Autodesk Fusion 360 part; units mm, degrees
note: some values were not read from the file. Set by a fixed rule: which sketch regions a step uses.
(part 2 of 2)
  constraint tangent L244 A250
  constraint tangent L243 A251
  constraint tangent L250 A251
  constraint tangent L251 A252
  constraint tangent L243 A252
  constraint tangent L242 A253
  constraint tangent L251 A253
  constraint tangent L242 A254
  constraint tangent L241 A254
  constraint tangent L241 A255
  constraint tangent L240 A255
  constraint tangent L240 A256
  constraint tangent L239 A256
  constraint tangent L239 A257
  constraint tangent L238 A257
  constraint perpendicular L104 L253
  constraint coincident L216 L253.start
  constraint tangent L229 A258
  constraint tangent L106 A259
  constraint tangent L253 A259
  constraint tangent L229 A260
  constraint tangent L106 A260
  constraint tangent L252 A261
  constraint tangent L252 A262
  measures "d1" diameter of A0
  measures "d2" diameter of A1
  measures "d3" diameter of A2
  measures "d4" diameter of A3
  measures "d5" diameter of A4
  measures "d9" diameter of A111
  measures "d12" diameter of A112
extrude "Extrude1" add sketch "mriya-bumper-fdm" along normal blind 10.5 contours L181 L182 L207 A214 L208 A215 L209 A216 L210 A217 L211 A218 L212 A219 L213 A220 L214 A221 L215 A222 L216 L217 A224 L218 A225 L219 A226 L220 A227 L221 A228 L222 A229 L223 A230 L224 A231 L225 A232 L226 A233 L227 A234 L228 A235 L230 L231 L232 L233 L234 L235 L236 L237 L238 L239 L240 L241 L242 L243 L244 L245 L246 L247 L248 L249 L250 L251 A236 A237 A239 A240 A241 A242 A243 A244 A245 A246 A247 A248 A249 A250 A251 A252 A253 A254 A255 A256 A257 makes body 1
extrude "Extrude2" add sketch "mriya-bumper-fdm" along normal blind 17 contours L181 L182 L216 A223 L217 L245 L246 A238 bodies 1
extrude "Extrude3" add sketch "mriya-bumper-fdm" along normal blind 2 from surface at 1.7 contours L106 L207 A214 L208 A215 L209 A216 L210 A217 L211 A218 L212 A219 L213 A220 L214 A221 L215 A222 L216 L217 A224 L218 A225 L219 A226 L220 A227 L221 A228 L222 A229 L223 A230 L224 A231 L225 A232 L226 A233 L227 A234 L228 A235 L229 L252 A258 A259 A260 A261 A262 | L106 L216 A223 L217 L229 A258 A259 A260 | L216 L252 A261 A262 | A114 | A115 | A116 | A117 bodies 1
extrude "Extrude6" add sketch "mriya-bumper-fdm" along normal blind 1 from surface at 14.3 contours L106 L216 A223 L217 L229 A258 A259 A260 bodies 1
extrude "Extrude12" add sketch "mriya-bumper-fdm" along normal blind 1 from surface at 7.7 contours L216 L252 A261 A262 bodies 1
sketch "power-switch" plane through (-4.4, 0, 0) normal (1, 0, 0) x (0, 1, 0)
  line L0 (1.7932, 0) -> (76.6932, 0)
  line L1 (76.6932, 0) -> (76.6932, 17)
  line L2 (76.6932, 17) -> (19.2932, 17)
  line L3 (19.2932, 17) -> (19.2932, 10.5)
  line L4 (19.2932, 10.5) -> (1.7932, 10.5)
  line L5 (1.7932, 10.5) -> (1.7932, 0)
  line L6 (25.6932, 5.4) -> (25.6932, 8.35)
  line L7 (36.0932, 5.4) -> (25.6932, 5.4)
  arc A0 (37.3932, 4.05) -> (37.7932, 4.45) centre (37.3932, 4.45) ccw
  arc A1 (24.3932, 9.7) -> (23.9932, 9.3) centre (24.3932, 9.3) ccw
  line L8 (23.9932, 4.45) -> (23.9932, 9.3)
  line L9 (25.6932, 8.35) -> (36.0932, 8.35)
  arc A2 (23.9932, 4.45) -> (24.3932, 4.05) centre (24.3932, 4.45) ccw
  line L10 (37.7932, 9.3) -> (37.7932, 4.45)
  line L11 (37.3932, 4.05) -> (24.3932, 4.05)
  line L12 (24.3932, 9.7) -> (37.3932, 9.7)
  line L13 (36.0932, 8.35) -> (36.0932, 5.4)
  arc A3 (37.7932, 9.3) -> (37.3932, 9.7) centre (37.3932, 9.3) ccw
  constraint perpendicular L6 L7
  constraint vertical L6
  constraint perpendicular L6 L9
  constraint vertical L13
  constraint tangent L12 A3
  constraint tangent L10 A3
  constraint tangent A0 L10
  constraint tangent A0 L11
  constraint tangent A2 L11
  constraint tangent L8 A2
  constraint tangent A1 L8
  constraint tangent A1 L12
extrude "Extrude8" cut sketch "power-switch" against normal blind 2.5 contours L6 L7 L9 L13 bodies 1
extrude "Extrude9" cut sketch "power-switch" against normal blind 1 contours A0 A1 L8 A2 L10 L11 L12 A3 bodies 1
chamfer "Chamfer13" distance 1.19 angle 40 8 edges at (-4.4, 30.8932, 9.7) (-4.4, 37.676, 9.5828) (-4.4, 37.7932, 6.875) (-4.4, 37.676, 4.1672) (-4.4, 30.8932, 4.05) (-4.4, 24.1104, 4.1672) (-4.4, 23.9932, 6.875) (-4.4, 24.1104, 9.5828) measured on face at (-4.4, 63.7265, 8.7667) measured on face at (-4.4, 63.7265, 8.7667) measured on face at (-4.4, 63.7265, 8.7667) measured on face at (-4.4, 63.7265, 8.7667) measured on face at (-4.4, 63.7265, 8.7667) measured on face at (-4.4, 63.7265, 8.7667) measured on face at (-4.4, 63.7265, 8.7667) measured on face at (-4.4, 63.7265, 8.7667) on bodies 1
chamfer "Chamfer14" distance 0.5 angle 45 4 edges at (-6.9, 30.8932, 5.4) (-6.9, 25.6932, 6.875) (-6.9, 30.8932, 8.35) (-6.9, 36.0932, 6.875) on bodies 1
sketch "usb-c" plane through (0, 80.6932, 0) normal (0, 1, 0) x (-1, 0, 0)
  line L0 (8.4, 0) -> (41.0674, 0)
  line L1 (41.0674, 0) -> (41.0674, 10.5)
  line L2 (41.0674, 10.5) -> (26, 10.5)
  line L3 (26, 10.5) -> (26, 17)
  line L4 (26, 17) -> (8.4, 17)
  line L5 (8.4, 17) -> (8.4, 0)
  line L6 (11.0002, 8.3) -> (11.0002, 12.9)
  line L7 (21.0002, 11.1) -> (21.0002, 10.1)
  line L8 (11.8003, 10.1) -> (11.8003, 11.1)
  arc A0 (11.4002, 13.3) -> (11.0002, 12.9) centre (11.4002, 12.9) ccw
  line L9 (11.4002, 13.3) -> (21.4002, 13.3)
  line L10 (21.8003, 12.9) -> (21.8003, 8.3)
  arc A1 (21.8003, 12.9) -> (21.4002, 13.3) centre (21.4002, 12.9) ccw
  arc A2 (21.4002, 7.9) -> (21.8002, 8.3) centre (21.4002, 8.3) ccw
  line L11 (13.1003, 12.4) -> (19.7002, 12.4)
  line L12 (19.7002, 8.8) -> (13.1003, 8.8)
  line L13 (21.4002, 7.9) -> (11.4002, 7.9)
  arc A3 (11.0002, 8.3) -> (11.4002, 7.9) centre (11.4002, 8.3) ccw
  arc A4 (13.1003, 12.4) -> (11.8003, 11.1) centre (13.1003, 11.1) ccw
  arc A5 (11.8003, 10.1) -> (13.1003, 8.8) centre (13.1003, 10.1) ccw
  arc A6 (21.0002, 11.1) -> (19.7002, 12.4) centre (19.7002, 11.1) ccw
  arc A7 (19.7002, 8.8) -> (21.0002, 10.1) centre (19.7002, 10.1) ccw
  constraint perpendicular L9 L10
  constraint perpendicular L6 L13
  constraint horizontal L13
  constraint perpendicular L10 L13
  constraint tangent A0 L9
  constraint tangent L6 A0
  constraint tangent L9 A1
  constraint tangent L10 A1
  constraint tangent L6 A3
  constraint tangent L13 A3
  constraint tangent A2 L13
  constraint tangent L10 A2
  constraint tangent L11 A4
  constraint tangent L8 A4
  constraint tangent L8 A5
  constraint tangent L12 A5
  constraint tangent L7 A6
  constraint tangent L11 A6
  constraint tangent L12 A7
  constraint tangent L7 A7
extrude "Extrude13" cut sketch "usb-c" against normal blind 2.5 contours L7 L8 L11 L12 A4 A5 A6 A7 bodies 1
extrude "Extrude14" cut sketch "usb-c" against normal blind 1 contours L6 A0 L9 L10 A1 A2 L13 A3 bodies 1
chamfer "Chamfer22" distance 1.19 angle 40 8 edges at (-16.4003, 80.6932, 13.3) (-21.6831, 80.6932, 13.1828) (-21.8003, 80.6932, 10.6) (-21.6831, 80.6932, 8.0172) (-16.4003, 80.6932, 7.9) (-11.1174, 80.6932, 8.0172) (-11.0003, 80.6932, 10.6) (-11.1174, 80.6932, 13.1828) measured on face at (-23.6457, 80.6932, 2.6354) measured on face at (-23.6457, 80.6932, 2.6354) measured on face at (-23.6457, 80.6932, 2.6354) measured on face at (-23.6457, 80.6932, 2.6354) measured on face at (-23.6457, 80.6932, 2.6354) measured on face at (-23.6457, 80.6932, 2.6354) measured on face at (-23.6457, 80.6932, 2.6354) measured on face at (-23.6457, 80.6932, 2.6354) on bodies 1
chamfer "Chamfer20" distance 0.599 angle 45 3 edges at (-14.85, 78.1932, 14.3) (-7.3979, 77.6953, 14.3) (-6.9, 58.2432, 14.3) on bodies 1
chamfer "Chamfer21" distance 0.6 angle 45 1 edges at (-6.9, 9.5932, 7.7) on bodies 1
chamfer "Chamfer17" distance 1 angle 45 90 edges at (-17.0879, -2.2068, 10.5) (-5.5716, -1.0352, 10.5) (-4.4, 10.5432, 10.5) (-33.5337, 80.6932, 10.5) (-41.4501, 80.7693, 10.5) (-42.3387, 81.5503, 10.5) (-43.8762, 82.7648, 10.5) (-51.4458, 82.9932, 10.5) (-58.2501, 83.0693, 10.5) (-60.2387, 84.9503, 10.5) (-62.8762, 87.2648, 10.5) (-73.4, 87.4932, 10.5) (-83.9238, 87.2648, 10.5) (-86.0613, 85.4503, 10.5) (-87.5499, 84.0693, 10.5) (-94.8542, 83.9932, 10.5) (-102.9238, 83.7648, 10.5) (-107.238, 79.7735, 10.5) (-111.0657, 76.1074, 10.5) (-116.2077, 75.9932, 10.5) (-121.9238, 75.7648, 10.5) (-123.4613, 74.5503, 10.5) (-124.3499, 73.7693, 10.5) (-131.5163, 73.6932, 10.5) (-141.1284, 72.5216, 10.5) (-142.3, 42.8932, 10.5) (-141.1284, 13.2648, 10.5) (-120.4728, 12.0932, 10.5) (-100.9235, 12.4357, 10.5) (-96.4155, 16.4593, 10.5) (-92.7186, 19.941, 10.5) (-84.5898, 20.0932, 10.5) (-75.7143, 19.6842, 10.5) (-70.5474, 11.3702, 10.5) (-65.1972, 2.8703, 10.5) (-56.0828, 2.3932, 10.5) (-48.3499, 2.3171, 10.5) (-47.4613, 1.5361, 10.5) (-45.9238, 0.3216, 10.5) (-37.2542, 0.0932, 10.5) (-29.3499, 0.0171, 10.5) (-28.4613, -0.7639, 10.5) (-26.9238, -1.9784, 10.5) (-17.0879, -2.2068, 0) (-26.9238, -1.9784, 0) (-28.4613, -0.7639, 0) (-29.3499, 0.0171, 0) (-37.2542, 0.0932, 0) (-45.9238, 0.3216, 0) (-47.4613, 1.5361, 0) (-48.3499, 2.3171, 0) (-56.0828, 2.3932, 0) (-65.1972, 2.8703, 0) (-70.5474, 11.3702, 0) (-75.7143, 19.6842, 0) (-84.5898, 20.0932, 0) (-92.7186, 19.941, 0) (-96.4155, 16.4593, 0) (-100.9235, 12.4357, 0) (-120.4728, 12.0932, 0) (-141.1284, 13.2648, 0) (-142.3, 42.8932, 0) (-141.1284, 72.5216, 0) (-131.5163, 73.6932, 0) (-124.3499, 73.7693, 0) (-123.4613, 74.5503, 0) (-121.9238, 75.7648, 0) (-116.2077, 75.9932, 0) (-111.0657, 76.1074, 0) (-107.238, 79.7735, 0) (-102.9238, 83.7648, 0) (-94.8542, 83.9932, 0) (-87.5499, 84.0693, 0) (-86.0613, 85.4503, 0) (-83.9238, 87.2648, 0) (-73.4, 87.4932, 0) (-62.8762, 87.2648, 0) (-60.2387, 84.9503, 0) (-58.2501, 83.0693, 0) (-51.4458, 82.9932, 0) (-43.8762, 82.7648, 0) (-42.3387, 81.5503, 0) (-41.4501, 80.7693, 0) (-24.7337, 80.6932, 0) (-5.5716, 79.5216, 0) (-4.4, 39.2432, 0) (-5.5716, -1.0352, 0) (-4.4, 47.9932, 17) (-5.5716, 79.5216, 17) (-17.2, 80.6932, 17) on bodies 1
fillet "Fillet29" radius 1.2 2 edges at (-4.4, 19.2932, 12.75) (-26, 80.6932, 12.75) on bodies 1
chamfer "Chamfer18" distance 1 angle 45 4 edges at (-6.25, 19.2932, 17) (-5.4996, 19.2974, 17) (-26, 78.8432, 17) (-25.9958, 79.5936, 17) on bodies 1
mirror "Mirror1" about plane through (0, 0, 0) normal (1, 0, 0) of bodies 1 makes body 2
named bodies: "Left", "Right"
